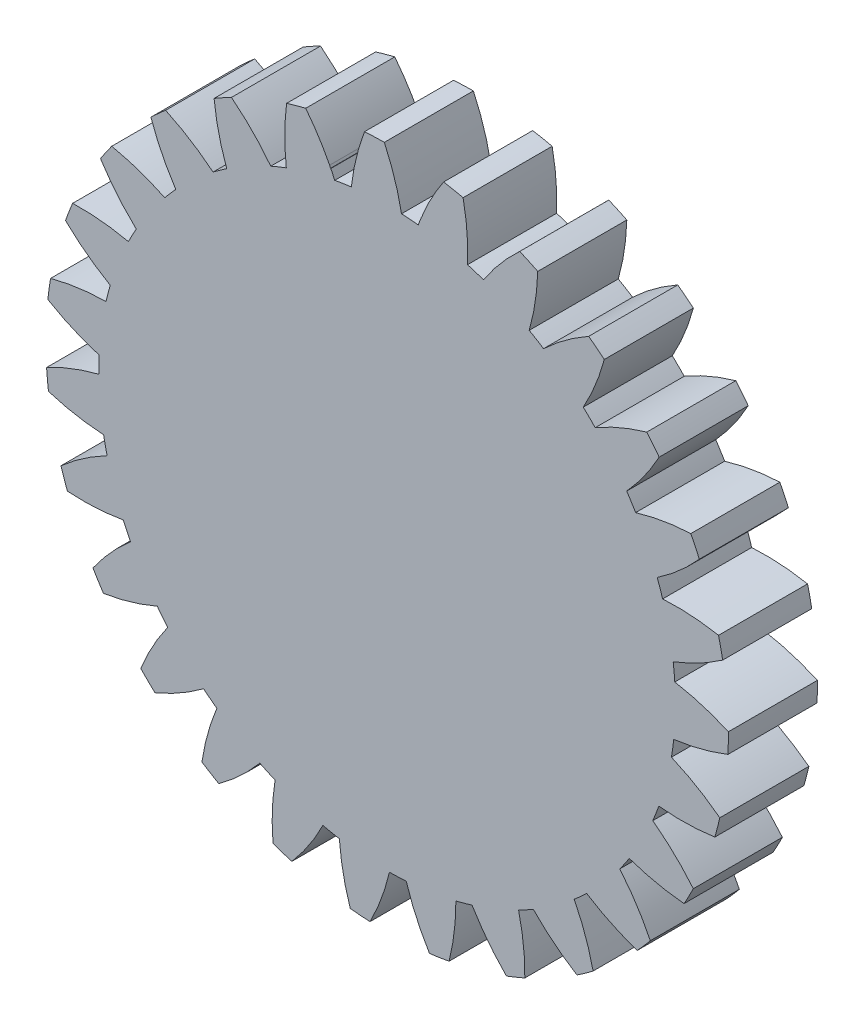
# Autodesk Inventor part: moon_gear_V1
Saved by Autodesk Inventor 2026 (Build 300175050, 175E)
## iProperties
Created: 2026-04-01
Part Number: moon_gear_V1
Material: Generic
Document SubType Name: Modeling
Designer: sniel
Density: 1 g/cm^3
Appearance: Default
Author: sniel
Autodesk Inventor part; units mm, degrees
ref_plane "YZ Plane" through (0, 0, 0) normal (1, 0, 0) x (0, 1, 0)
ref_plane "XZ Plane" through (0, 0, 0) normal (0, 1, 0) x (-1, 0, 0)
ref_plane "XY Plane" through (0, 0, 0) normal (0, 0, 1) x (1, 0, 0)
sketch "Sketch1" plane through (0, 0, 0) normal (0, 0, 1) x (1, 0, 0)
  arc A0 (-3.2265, 16.5156) -> (-4.5709, 18.6086) centre (-14.4821, 10.7637) ccw
  arc A1 (-3.181, 16.384) -> (-3.2265, 16.5156) centre (-21.5154, 10.1188) ccw
  arc A2 (-3.1609, 16.3854) -> (-3.181, 16.384) centre (2.6244, -70.4313) ccw
  arc A3 (-2.941, 15.919) -> (-3.1609, 16.3854) centre (-14.4821, 10.7637) ccw
  arc A4 (-2.0104, 16.0631) -> (-2.941, 15.919) centre (0, 0) ccw
  arc A5 (-1.2701, 19.1197) -> (-2.0104, 16.0631) centre (10.5492, 14.6391) ccw
  arc A6 (-0.1563, 19.1612) -> (-1.2701, 19.1197) centre (0, 0) ccw
  arc A7 (0.8094, 16.1682) -> (-0.1563, 19.1612) centre (-11.6094, 13.8134) ccw
  arc A8 (1.7482, 16.0938) -> (0.8094, 16.1682) centre (0, 0) ccw
  arc A9 (1.9327, 16.5752) -> (1.7482, 16.0938) centre (13.6409, 11.8117) ccw
  arc A10 (1.9528, 16.5753) -> (1.9327, 16.5752) centre (2.6244, -70.4313) ccw
  arc A11 (1.9884, 16.71) -> (1.9528, 16.5753) centre (20.7027, 11.6919) ccw
  arc A12 (3.1734, 18.8972) -> (1.9884, 16.71) centre (13.6409, 11.8117) ccw
  arc A13 (4.2668, 18.6807) -> (3.1734, 18.8972) centre (0, 0) ccw
  arc A14 (4.5162, 15.5457) -> (4.2668, 18.6807) centre (-8.1109, 16.1184) ccw
  arc A15 (5.4125, 15.2568) -> (4.5162, 15.5457) centre (0, 0) ccw
  arc A16 (7.4458, 17.656) -> (5.4125, 15.2568) centre (15.9972, 8.3475) ccw
  arc A17 (8.4599, 17.1932) -> (7.4458, 17.656) centre (0, 0) ccw
  arc A18 (7.9796, 14.0851) -> (8.4599, 17.1932) centre (-4.1751, 17.5544) ccw
  arc A19 (8.7851, 13.5973) -> (7.9796, 14.0851) centre (0, 0) ccw
  arc A20 (11.3169, 15.4629) -> (8.7851, 13.5973) centre (17.491, 4.4333) ccw
  arc A21 (12.1968, 14.7788) -> (11.3169, 15.4629) centre (0, 0) ccw
  arc A22 (11.0128, 11.8652) -> (12.1968, 14.7788) centre (-0.0143, 18.0441) ccw
  arc A23 (11.684, 11.2048) -> (11.0128, 11.8652) centre (0, 0) ccw
  arc A24 (14.5778, 12.4363) -> (11.684, 11.2048) centre (18.0419, 0.2801) ccw
  arc A25 (15.2763, 11.5676) -> (14.5778, 12.4363) centre (0, 0) ccw
  arc A26 (13.4522, 9.0057) -> (15.2763, 11.5676) centre (4.1474, 17.561) ccw
  arc A27 (13.9531, 8.2083) -> (13.4522, 9.0057) centre (0, 0) ccw
  arc A28 (17.0529, 8.7392) -> (13.9531, 8.2083) centre (17.6202, -3.8882) ccw
  arc A29 (17.5322, 7.7329) -> (17.0529, 8.7392) centre (0, 0) ccw
  arc A30 (15.1665, 5.6607) -> (17.5322, 7.7329) centre (8.0854, 16.1312) ccw
  arc A31 (15.47, 4.7692) -> (15.1665, 5.6607) centre (0, 0) ccw
  arc A32 (18.6086, 4.5709) -> (15.47, 4.7692) centre (16.2485, -7.8469) ccw
  arc A33 (18.8429, 3.4812) -> (18.6086, 4.5709) centre (0, 0) ccw
  arc A34 (16.0631, 2.0104) -> (18.8429, 3.4812) centre (11.5876, 13.8317) ccw
  arc A35 (16.1528, 1.0731) -> (16.0631, 2.0104) centre (0, 0) ccw
  arc A36 (19.1612, 0.1563) -> (16.1528, 1.0731) centre (14.0009, -11.3826) ccw
  arc A37 (19.1378, -0.9581) -> (19.1612, 0.1563) centre (0, 0) ccw
  arc A38 (16.0938, -1.7482) -> (19.1378, -0.9581) centre (14.4651, 10.7866) ccw
  arc A39 (15.9649, -2.681) -> (16.0938, -1.7482) centre (0, 0) ccw
  arc A40 (18.6807, -4.2668) -> (15.9649, -2.681) centre (10.9985, -14.3046) ccw
  arc A41 (18.401, -5.3458) -> (18.6807, -4.2668) centre (0, 0) ccw
  arc A42 (15.2568, -5.4125) -> (18.401, -5.3458) centre (16.5627, 7.16) ccw
  arc A43 (14.9163, -6.2905) -> (15.2568, -5.4125) centre (0, 0) ccw
  arc A44 (17.1932, -8.4599) -> (14.9163, -6.2905) centre (7.4032, -16.4555) ccw
  arc A45 (16.6722, -9.4452) -> (17.1932, -8.4599) centre (0, 0) ccw
  arc A46 (13.5973, -8.7851) -> (16.6722, -9.4452) centre (17.7675, 3.1474) ccw
  arc A47 (13.0635, -9.5608) -> (13.5973, -8.7851) centre (0, 0) ccw
  arc A48 (14.7788, -12.1968) -> (13.0635, -9.5608) centre (3.4088, -17.7192) ccw
  arc A49 (14.0446, -13.0355) -> (14.7788, -12.1968) centre (0, 0) ccw
  arc A50 (11.2048, -11.684) -> (14.0446, -13.0355) centre (18.0144, -1.0349) ccw
  arc A51 (10.5065, -12.3158) -> (11.2048, -11.684) centre (0, 0) ccw
  arc A52 (11.5676, -15.2763) -> (10.5065, -12.3158) centre (-0.7695, -18.0277) ccw
  arc A53 (10.6598, -15.923) -> (11.5676, -15.2763) centre (0, 0) ccw
  arc A54 (8.2083, -13.9531) -> (10.6598, -15.923) centre (17.2901, -5.1614) ccw
  arc A55 (7.3831, -14.4068) -> (8.2083, -13.9531) centre (0, 0) ccw
  arc A56 (7.7329, -17.5322) -> (7.3831, -14.4068) centre (-4.9062, -17.3643) ccw
  arc A57 (6.7004, -17.9522) -> (7.7329, -17.5322) centre (0, 0) ccw
  arc A58 (4.7692, -15.47) -> (6.7004, -17.9522) centre (15.6338, -9.0097) ccw
  arc A59 (3.8617, -15.7211) -> (4.7692, -15.47) centre (0, 0) ccw
  arc A60 (3.4812, -18.8429) -> (3.8617, -15.7211) centre (-8.7784, -15.7648) ccw
  arc A61 (2.3797, -19.0135) -> (3.4812, -18.8429) centre (0, 0) ccw
  arc A62 (1.0731, -16.1528) -> (2.3797, -19.0135) centre (13.1346, -12.3722) ccw
  arc A63 (0.132, -16.1879) -> (1.0731, -16.1528) centre (0, 0) ccw
  arc A64 (-0.9581, -19.1378) -> (0.132, -16.1879) centre (-12.1774, -13.3154) ccw
  arc A65 (-2.0692, -19.0497) -> (-0.9581, -19.1378) centre (0, 0) ccw
  arc A66 (-2.681, -15.9649) -> (-2.0692, -19.0497) centre (9.9273, -15.0678) ccw
  arc A67 (-3.6047, -15.782) -> (-2.681, -15.9649) centre (0, 0) ccw
  arc A68 (-5.3458, -18.401) -> (-3.6047, -15.782) centre (-14.9199, -10.1482) ccw
  arc A69 (-6.4066, -18.0591) -> (-5.3458, -18.401) centre (0, 0) ccw
  arc A70 (-6.2905, -14.9163) -> (-6.4066, -18.0591) centre (6.1848, -16.951) ccw
  arc A71 (-7.1471, -14.5253) -> (-6.2905, -14.9163) centre (0, 0) ccw
  arc A72 (-9.4452, -16.6722) -> (-7.1471, -14.5253) centre (-16.8581, -6.4339) ccw
  arc A73 (-10.3987, -16.0948) -> (-9.4452, -16.6722) centre (0, 0) ccw
  arc A74 (-9.5608, -13.0635) -> (-10.3987, -16.0948) centre (2.109, -17.9204) ccw
  arc A75 (-10.3042, -12.4855) -> (-9.5608, -13.0635) centre (0, 0) ccw
  arc A76 (-13.0355, -14.0446) -> (-10.3042, -12.4855) centre (-17.8874, -2.3727) ccw
  arc A77 (-13.8301, -13.2629) -> (-13.0355, -14.0446) centre (0, 0) ccw
  arc A78 (-12.3158, -10.5065) -> (-13.8301, -13.2629) centre (-2.0806, -17.9237) ccw
  arc A79 (-12.9058, -9.7726) -> (-12.3158, -10.5065) centre (0, 0) ccw
  arc A80 (-15.923, -10.6598) -> (-12.9058, -9.7726) centre (-17.9524, 1.8164) ccw
  arc A81 (-16.5159, -9.7159) -> (-15.923, -10.6598) centre (0, 0) ccw
  arc A82 (-14.4068, -7.3831) -> (-16.5159, -9.7159) centre (-6.158, -16.9608) ccw
  arc A83 (-14.8117, -6.5329) -> (-14.4068, -7.3831) centre (0, 0) ccw
  arc A84 (-17.9522, -6.7004) -> (-14.8117, -6.5329) centre (-17.0497, 5.9075) ccw
  arc A85 (-18.3114, -5.6452) -> (-17.9522, -6.7004) centre (0, 0) ccw
  arc A86 (-15.7211, -3.8617) -> (-18.3114, -5.6452) centre (-9.9035, -15.0835) ccw
  arc A87 (-15.919, -2.941) -> (-15.7211, -3.8617) centre (0, 0) ccw
  arc A88 (-19.0135, -2.3797) -> (-15.919, -2.941) centre (-15.2277, 9.6802) ccw
  arc A89 (-19.1197, -1.2701) -> (-19.0135, -2.3797) centre (0, 0) ccw
  arc A90 (-16.1879, -0.132) -> (-19.1197, -1.2701) centre (-13.115, -12.393) ccw
  arc A91 (-16.1682, 0.8094) -> (-16.1879, -0.132) centre (0, 0) ccw
  arc A92 (-19.0497, 2.0692) -> (-16.1682, 0.8094) centre (-12.5848, 12.931) ccw
  arc A93 (-18.8972, 3.1734) -> (-19.0497, 2.0692) centre (0, 0) ccw
  arc A94 (-15.782, 3.6047) -> (-18.8972, 3.1734) centre (-15.6195, -9.0344) ccw
  arc A95 (-15.5457, 4.5162) -> (-15.782, 3.6047) centre (0, 0) ccw
  arc A96 (-18.0591, 6.4066) -> (-15.5457, 4.5162) centre (-9.2635, 15.4847) ccw
  arc A97 (-17.656, 7.4458) -> (-18.0591, 6.4066) centre (0, 0) ccw
  arc A98 (-14.5253, 7.1471) -> (-17.656, 7.4458) centre (-17.282, -5.1888) ccw
  arc A99 (-14.0851, 7.9796) -> (-14.5253, 7.1471) centre (0, 0) ccw
  arc A100 (-16.0948, 10.3987) -> (-14.0851, 7.9796) centre (-5.4428, 17.2036) ccw
  arc A101 (-15.4629, 11.3169) -> (-16.0948, 10.3987) centre (0, 0) ccw
  arc A102 (-12.4855, 10.3042) -> (-15.4629, 11.3169) centre (-18.0127, -1.0634) ccw
  arc A103 (-11.8652, 11.0128) -> (-12.4855, 10.3042) centre (0, 0) ccw
  arc A104 (-13.2629, 13.8301) -> (-11.8652, 11.0128) centre (-1.3286, 17.9951) ccw
  arc A105 (-12.4363, 14.5778) -> (-13.2629, 13.8301) centre (0, 0) ccw
  arc A106 (-9.7726, 12.9058) -> (-12.4363, 14.5778) centre (-17.7724, 3.1193) ccw
  arc A107 (-9.0057, 13.4522) -> (-9.7726, 12.9058) centre (0, 0) ccw
  arc A108 (-9.7159, 16.5159) -> (-9.0057, 13.4522) centre (2.8571, 17.8165) ccw
  arc A109 (-8.7392, 17.0529) -> (-9.7159, 16.5159) centre (0, 0) ccw
  arc A110 (-6.5329, 14.8117) -> (-8.7392, 17.0529) centre (-16.574, 7.1338) ccw
  arc A111 (-5.6607, 15.1665) -> (-6.5329, 14.8117) centre (0, 0) ccw
  arc A112 (-5.6452, 18.3114) -> (-5.6607, 15.1665) centre (6.8889, 16.6773) ccw
  arc A113 (-4.5709, 18.6086) -> (-5.6452, 18.3114) centre (0, 0) ccw
  point P0 (0, 0)
  constraints: 228 point on circle, 114 centre point
extrude "Extrusion1" add sketch "Sketch1" along normal blind 5
sketch "Sketch2" plane through (0, 0, 0) normal (0, 0, -1) x (-1, 0, 0)
  circle A0 centre (0, 0) radius 4.75
  dimension "d2" = 9.5
  constraints: 1 centre point, 1 coincident
  measures "d2" diameter of A0
extrude "Extrusion2" add sketch "Sketch2" along normal blind 8
body "Solid1"
